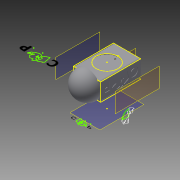
# Autodesk Inventor part: Pieza2
Saved by Autodesk Inventor 2013 (Build 170138000, 138)
## iProperties
Created: 2014-07-03
Part Number: Pieza2
Material: Genérico
Document SubType Name: Chapa
Designer: Administrador
Density: 1 g/cm^3
Sheet Metal Rule: Por defecto_mm
Author: Administrador
Autodesk Inventor part; units mm, degrees
ref_plane "YZ Plane" through (0, 0, 0) normal (1, 0, 0) x (0, 1, 0)
ref_plane "XZ Plane" through (0, 0, 0) normal (0, 1, 0) x (-1, 0, 0)
ref_plane "XY Plane" through (0, 0, 0) normal (0, 0, 1) x (1, 0, 0)
sketch "Boceto1" plane through (0, 0, 0) normal (0, 0, 1) x (1, 0, 0)
  line L0 (-17, 25) -> (17, 25)
  line L1 (17, 25) -> (17, -25)
  line L2 (17, -25) -> (-17, -25)
  line L3 (-17, -25) -> (-17, 25)
  line L4 (17, 25) -> (-17, -25) construction
  line L5 (-17, 25) -> (17, -25) construction
  point P0 (0, 0)
  point P1 (0, 0)
  dimension "d0" = 34
  dimension "d1" = 50
  constraints: 12 end point, 2 midpoint, 2 parallel, 1 coincident, 1 horizontal, 1 perpendicular
  measures "d0" distance of L1.end L2.end
  measures "d1" distance of L0.end L1.end
extrude "Extrusión1" add sketch "Boceto1" along normal mid plane 22
sketch "Boceto2" plane through (-17, -25, 11) normal (0, -1, 0) x (1, 0, 0)
  line L0 (34, 0) -> (34, -22) projected
  line L1 (0, 0) -> (34, 0) projected
  line L2 (0, 0) -> (0, -22) projected
  line L3 (34, -22) -> (0, -22) projected
  line L4 (32, 0) -> (0, -22) construction
  line L5 (0, 0) -> (32, -22) construction
  point P0 (17, -11)
  constraints: 4 end point
ref_plane "Plano de trabajo1" through (1, -25, 11) normal (1, 0, 0) x (0, 0, -1)
sketch "Boceto4" plane through (1, -25, 11) normal (1, 0, 0) x (0, 0, -1)
  arc A0 (62.0687, 50.9812) -> (70.5687, 42.4812) centre (70.5687, 50.9812) ccw
  arc A1 (63.0687, 50.9812) -> (70.5687, 43.4812) centre (70.5687, 50.9812) ccw
  line L0 (70.5687, 50.9812) -> (62.0687, 50.9812)
  line L1 (70.5687, 50.9812) -> (70.5687, 42.4812)
  point P0 (11, 25)
  dimension "d19" = 17
  dimension "d20" = 15
  constraints: 4 end point, 4 point on circle, 2 centre point, 2 point on line
  measures "d19" diameter of A0
  measures "d20" diameter of A1
ref_plane "Plano de trabajo2" through (0, -25, 11) normal (1, 0, 0) x (0, 0, -1)
sketch "Boceto5" plane through (0, -25, 11) normal (1, 0, 0) x (0, 0, -1)
  arc A0 (11, -16.622) -> (28, 0.378) centre (11, 0.378) ccw
  arc A1 (11, -14.622) -> (26, 0.378) centre (11, 0.378) ccw
  line L0 (11, 0.378) -> (11, -19.6766)
  line L1 (11, 0.378) -> (38.473, 0.378)
  point P0 (11, 25)
  dimension "d25" = 34
  dimension "d26" = 30
  constraints: 4 end point, 4 point on circle, 4 point on line, 2 centre point
  measures "d25" diameter of A0
  measures "d26" diameter of A1
revolve "Revolución2" add sketch "Boceto5" angle 360 about axis through (0, -24.622, 0) along (0, -1, 0) contours L0 A1 L1 A0
shell "Vaciado1" thickness 2 removed faces 1 at (5.6667, 25, 3.6667)
sketch "Boceto6" plane through (0, 0, -11) normal (0, 0, -1) x (-1, 0, 0)
  arc A0 (-0.9993, 13.463) -> (0.9993, 13.463) centre (0, 0) ccw
  arc A1 (0.9993, 13.463) -> (-0.9993, 13.463) centre (0, 13.4998) ccw
  dimension "d29" = 27
  dimension "d34" = 2
  constraints: 4 point on circle, 2 centre point
  measures "d29" diameter of A0
  measures "d34" diameter of A1
extrude "Extrusión2" cut sketch "Boceto6" against normal blind 1
sketch "Boceto7" plane through (0, 0, 11) normal (0, 0, 1) x (1, 0, 0)
  arc A0 (-0.9993, 13.463) -> (0.9993, 13.463) centre (0, 0) ccw projected
  arc A1 (0.9993, 13.463) -> (-0.9993, 13.463) centre (0, 13.4998) ccw projected
extrude "Extrusión3" cut sketch "Boceto7" against normal blind 1
hole "Hole2" at (0.5516, 9.7228, -10) direction (0, 0, 1) diameter 2 end through all
sketch "Boceto8" plane through (0, 0, -11) normal (0, 0, -1) x (-1, 0, 0)
  arc A0 (-0.9993, 13.463) -> (0.9993, 13.463) centre (0, 0) ccw projected
  arc A1 (0.9993, 13.463) -> (-0.9993, 13.463) centre (0, 13.4998) ccw projected
  arc A2 (-12.9615, -24.622) -> (-12.956, -25) centre (0, -24.622) ccw projected
  line L0 (-12.9615, -24.622) -> (-10.198, -24.622) projected
  arc A3 (-10.198, -24.622) -> (-10.191, -25) centre (0, -24.622) ccw projected
  line L1 (-10.191, -25) -> (10.191, -25) projected
  arc A4 (10.191, -25) -> (10.198, -24.622) centre (0, -24.622) ccw projected
  line L2 (10.198, -24.622) -> (12.9615, -24.622) projected
  arc A5 (12.956, -25) -> (12.9615, -24.622) centre (0, -24.622) ccw projected
  line L3 (12.956, -25) -> (17, -25) projected
  line L4 (17, -25) -> (17, 25) projected
  line L5 (17, 25) -> (-17, 25) projected
  line L6 (-17, 25) -> (-17, -25) projected
  line L7 (-17, -25) -> (-12.956, -25) projected
sketch "Boceto9" plane through (-15, -23, -9) normal (0, 1, 0) x (1, 0, 0)
  arc A0 (27.9615, 2) -> (2.0385, 2) centre (15, -9) ccw projected
  arc A1 (2.0385, -20) -> (27.9615, -20) centre (15, -9) ccw projected
  circle A2 centre (15, -9) radius 4.05
  point P0 (15, -9)
  dimension "d57" = 8.1
  constraints: 1 centre point
  measures "d57" diameter of A2
extrude "Extrusión4" cut sketch "Boceto9" against normal blind 1
ref_plane "Plano de trabajo3" through (-36.25, -25, 11) normal (-1, 0, 0) x (0, 0, 1)
sketch "Boceto10" plane through (-36.25, -25, 11) normal (-1, 0, 0) x (0, 0, 1)
  line L0 (-17.7826, 33.8086) -> (-14.5363, 27.7029)
  line L1 (-13.9978, 26.6902) -> (-13.9974, 26.6894)
  line L2 (-12.2413, 28.1075) -> (-14.5363, 27.7029)
  line L3 (-11.5169, 27.1267) -> (-14.0003, 26.6889)
  ellipse E0 centre (-9.6601, 27.8136) end of major axis (-7.0347, 26.2904) minor radius 1.6776 (-8.1725, 28.825) -> (-12.2413, 28.1075) ccw
  ellipse E1 centre (-10.8449, 20.7604) end of major axis (-14.0003, 26.6889) minor radius 3.4629 (-13.9978, 26.6902) -> (-7.6919, 14.8305) ccw
  line L4 (-5.4899, 29.298) -> (-8.1725, 28.825)
  line L5 (-4.9509, 28.2844) -> (-7.2786, 27.874)
  line L6 (-4.9509, 28.2844) -> (-3.2498, 25.0851)
  line L7 (-17.7826, 33.8086) -> (-8.7364, 35.4037)
  line L8 (-8.7364, 35.4037) -> (-5.4899, 29.298)
  line L9 (-7.3044, 36.4363) -> (-7.3044, 32.7107) construction
  line L10 (-17.7826, 33.8086) -> (-17.7826, 24.6228) construction
  line L11 (-17.7826, 33.8086) -> (-17.7826, 13.3894) construction
  ellipse E2 centre (-9.6601, 27.8136) end of major axis (-7.0347, 26.2904) minor radius 1.6776 (-11.5169, 27.1267) -> (-7.2786, 27.874) ccw
  ellipse E3 centre (-9.6601, 24.5302) end of major axis (-6.0844, 19.1017) minor radius 3.6119 (-10.4961, 20.1047) -> (-5.6523, 24.6615) ccw
  ellipse E4 centre (-9.0943, 17.4675) end of major axis (-10.4964, 20.1046) minor radius 1.3012 (-10.4961, 20.1047) -> (-7.6919, 14.8305) ccw
  line L12 (-10.4964, 20.1046) -> (-7.6922, 14.8304) construction
  line L13 (-3.2498, 25.0851) -> (-5.6523, 24.6615)
  line L14 (-7.6615, 46.9866) -> (-7.6615, 19.6947) construction
  line L15 (-7.6615, 19.6947) -> (-18.0504, 19.6947) construction
  line L16 (-18.0504, 19.6947) -> (-18.0504, 46.9866) construction
  line L17 (-18.0504, 46.9866) -> (-7.6615, 46.9866) construction
  line L18 (-7.8627, 12.5769) -> (-7.8627, 3.5412) construction
  line L19 (-7.8627, 3.5412) -> (-17.8627, 3.5412) construction
  line L20 (-17.8627, 3.5412) -> (-17.8627, 12.5769) construction
  line L21 (-17.8627, 12.5769) -> (-7.8627, 12.5769) construction
  spline S0 degree 2 poles (-18.0504, 41.6381) (-18.0504, 43.891) (-15.3276, 46.5328) (-12.864, 46.5328) knots 0 0 0 1 2 2 2
  spline S1 degree 2 poles (-12.864, 46.5328) (-10.4897, 46.5328) (-7.6615, 43.8828) (-7.6615, 41.63) knots 0 0 0 1 2 2 2
  spline S2 degree 2 poles (-7.6615, 41.63) (-7.6615, 41.0384) (-7.7992, 40.0822) (-7.9127, 39.6446) knots 0 0 0 1 2 2 2
  spline S3 degree 2 poles (-7.9127, 39.6446) (-8.018, 39.3042) (-8.3665, 38.502) (-8.4961, 38.2508) knots 0 0 0 1 2 2 2
  line L22 (-8.4961, 38.2508) -> (-10.8786, 38.2508)
  line L23 (-10.8786, 38.2508) -> (-10.8786, 38.502)
  spline S4 degree 2 poles (-10.8786, 38.502) (-10.7166, 38.6884) (-10.2627, 39.2394) (-10.0521, 39.5879) knots 0 0 0 1 2 2 2
  spline S5 degree 2 poles (-10.0521, 39.5879) (-9.8333, 39.9363) (-9.5334, 40.771) (-9.5334, 41.2329) knots 0 0 0 1 2 2 2
  spline S6 degree 2 poles (-9.5334, 41.2329) (-9.5334, 41.7759) (-9.8738, 42.6754) (-10.3033, 43.0887) knots 0 0 0 1 2 2 2
  spline S7 degree 2 poles (-10.3033, 43.0887) (-10.6841, 43.4615) (-11.9888, 43.9396) (-12.8721, 43.9396) knots 0 0 0 1 2 2 2
  spline S8 degree 2 poles (-12.8721, 43.9396) (-13.8041, 43.9396) (-15.0764, 43.4452) (-15.4653, 43.0401) knots 0 0 0 1 2 2 2
  spline S9 degree 2 poles (-15.4653, 43.0401) (-15.8462, 42.6511) (-16.1785, 41.6948) (-16.1785, 41.2167) knots 0 0 0 1 2 2 2
  spline S10 degree 2 poles (-16.1785, 41.2167) (-16.1785, 40.7224) (-15.8462, 39.8229) (-15.6436, 39.5149) knots 0 0 0 1 2 2 2
  spline S11 degree 2 poles (-15.6436, 39.5149) (-15.441, 39.1746) (-15.0115, 38.664) (-14.8414, 38.4777) knots 0 0 0 1 2 2 2
  line L24 (-14.8414, 38.4777) -> (-14.8414, 38.2508)
  line L25 (-14.8414, 38.2508) -> (-17.1914, 38.2508)
  spline S12 degree 2 poles (-17.1914, 38.2508) (-17.3211, 38.5263) (-17.6452, 39.2475) (-17.7587, 39.6365) knots 0 0 0 1 2 2 2
  spline S13 degree 2 poles (-17.7587, 39.6365) (-17.9046, 40.1065) (-18.0504, 40.925) (-18.0504, 41.6381) knots 0 0 0 1 2 2 2
  spline S14 degree 2 poles (-11.015, 3.8492) (-11.7119, 3.8492) (-12.9761, 4.2949) (-13.3975, 4.7082) knots 0 0 0 1 2 2 2
  spline S15 degree 2 poles (-13.3975, 4.7082) (-13.6649, 4.9594) (-14.1025, 5.5753) (-14.2565, 5.9399) knots 0 0 0 1 2 2 2
  spline S16 degree 2 poles (-14.2565, 5.9399) (-14.4105, 6.3127) (-14.5888, 7.1798) (-14.5888, 7.7147) knots 0 0 0 1 2 2 2
  line L26 (-14.5888, 7.7147) -> (-14.5888, 9.0275)
  line L27 (-14.5888, 9.0275) -> (-17.8627, 9.0275)
  line L28 (-17.8627, 9.0275) -> (-17.8627, 11.5396)
  line L29 (-17.8627, 11.5396) -> (-7.8627, 11.5396)
  line L30 (-7.8627, 11.5396) -> (-7.8627, 7.6579)
  spline S17 degree 2 poles (-7.8627, 7.6579) (-7.8627, 6.7989) (-8.1787, 5.5429) (-8.5191, 5.0323) knots 0 0 0 1 2 2 2
  spline S18 degree 2 poles (-8.5191, 5.0323) (-8.9, 4.4651) (-10.1479, 3.8492) (-11.015, 3.8492) knots 0 0 0 1 2 2 2
  spline S19 degree 2 poles (-11.0799, 6.4262) (-10.6504, 6.4262) (-10.0426, 6.8313) (-9.9291, 7.1069) knots 0 0 0 1 2 2 2
  spline S20 degree 2 poles (-9.9291, 7.1069) (-9.7752, 7.4634) (-9.7265, 8.1117) (-9.7265, 8.6709) knots 0 0 0 1 2 2 2
  line L31 (-9.7265, 8.6709) -> (-9.7265, 9.0275)
  line L32 (-9.7265, 9.0275) -> (-12.7249, 9.0275)
  line L33 (-12.7249, 9.0275) -> (-12.7249, 8.8492)
  spline S21 degree 2 poles (-12.7249, 8.8492) (-12.7249, 8.5007) (-12.7087, 7.8686) (-12.6682, 7.6336) knots 0 0 0 1 2 2 2
  spline S22 degree 2 poles (-12.6682, 7.6336) (-12.6358, 7.431) (-12.4413, 6.9853) (-12.3197, 6.8638) knots 0 0 0 1 2 2 2
  spline S23 degree 2 poles (-12.3197, 6.8638) (-12.0766, 6.6044) (-11.5337, 6.4262) (-11.0799, 6.4262) knots 0 0 0 1 2 2 2
  point P0 (-11, 25)
  dimension "d63" = 100
  constraints: 28 end point, 2 point on line, 1 equal length, 26 other
  measures "d63" angle of L10 L7
emboss "Repujado2" sketch "Boceto10" operation cut depth 0.5 direction (1, 0, 0)
ref_plane "Plano de trabajo4" through (37.75, -25, 11) normal (1, 0, 0) x (0, 0, -1)
sketch "Boceto11" plane through (37.75, -25, 11) normal (1, 0, 0) x (0, 0, -1)
  line L0 (17.9928, 28.2607) -> (15.6652, 27.8504)
  line L1 (17.4539, 29.2744) -> (14.7713, 28.8014)
  line L2 (14.2074, 35.3801) -> (17.4539, 29.2744)
  ellipse E0 centre (13.2836, 27.79) end of major axis (15.909, 26.2668) minor radius 1.6776 (11.4269, 27.1031) -> (15.6652, 27.8504) ccw
  ellipse E1 centre (13.2836, 27.79) end of major axis (15.909, 26.2668) minor radius 1.6776 (14.7713, 28.8014) -> (10.7025, 28.0839) ccw
  line L3 (15.6393, 36.4127) -> (15.6393, 32.6871) construction
  line L4 (11.4269, 27.1031) -> (8.9435, 26.6653)
  line L5 (10.7025, 28.0839) -> (8.4075, 27.6792)
  line L6 (5.1612, 33.785) -> (8.4075, 27.6792)
  line L7 (5.1612, 33.785) -> (14.2074, 35.3801)
  line L8 (15.2823, 19.6711) -> (4.8933, 19.6711) construction
  line L9 (4.8933, 46.9629) -> (15.2823, 46.9629) construction
  line L10 (15.2823, 46.9629) -> (15.2823, 19.6711) construction
  line L11 (4.8933, 19.6711) -> (4.8933, 46.9629) construction
  line L12 (8.9459, 26.6666) -> (8.9464, 26.6658)
  line L13 (17.9928, 28.2607) -> (19.6939, 25.0615)
  line L14 (19.6939, 25.0615) -> (17.2915, 24.6379)
  ellipse E2 centre (13.2836, 24.5066) end of major axis (16.8594, 19.0781) minor radius 3.6119 (12.4477, 20.0811) -> (17.2915, 24.6379) ccw
  line L15 (12.4474, 20.0809) -> (15.2516, 14.8068) construction
  ellipse E3 centre (13.8495, 17.4439) end of major axis (12.4474, 20.0809) minor radius 1.3012 (12.4477, 20.0811) -> (15.2518, 14.8069) ccw
  ellipse E4 centre (12.0989, 20.7367) end of major axis (8.9435, 26.6653) minor radius 3.4628 (8.9459, 26.6666) -> (15.2518, 14.8069) ccw
  line L16 (5.0811, 12.5533) -> (15.0811, 12.5533) construction
  line L17 (15.0811, 12.5533) -> (15.0811, 3.5176) construction
  line L18 (15.0811, 3.5176) -> (5.0811, 3.5176) construction
  line L19 (5.0811, 3.5176) -> (5.0811, 12.5533) construction
  spline S0 degree 2 poles (4.8933, 41.6145) (4.8933, 43.8673) (7.6162, 46.5091) (10.0797, 46.5091) knots 0 0 0 1 2 2 2
  spline S1 degree 2 poles (10.0797, 46.5091) (12.4541, 46.5091) (15.2823, 43.8592) (15.2823, 41.6064) knots 0 0 0 1 2 2 2
  spline S2 degree 2 poles (15.2823, 41.6064) (15.2823, 41.0148) (15.1446, 40.0586) (15.0311, 39.621) knots 0 0 0 1 2 2 2
  spline S3 degree 2 poles (15.0311, 39.621) (14.9258, 39.2806) (14.5773, 38.4783) (14.4476, 38.2271) knots 0 0 0 1 2 2 2
  line L20 (14.4476, 38.2271) -> (12.0651, 38.2271)
  line L21 (12.0651, 38.2271) -> (12.0651, 38.4783)
  spline S4 degree 2 poles (12.0651, 38.4783) (12.2272, 38.6647) (12.681, 39.2158) (12.8917, 39.5642) knots 0 0 0 1 2 2 2
  spline S5 degree 2 poles (12.8917, 39.5642) (13.1105, 39.9127) (13.4104, 40.7474) (13.4104, 41.2093) knots 0 0 0 1 2 2 2
  spline S6 degree 2 poles (13.4104, 41.2093) (13.4104, 41.7522) (13.07, 42.6518) (12.6405, 43.0651) knots 0 0 0 1 2 2 2
  spline S7 degree 2 poles (12.6405, 43.0651) (12.2596, 43.4378) (10.9549, 43.9159) (10.0716, 43.9159) knots 0 0 0 1 2 2 2
  spline S8 degree 2 poles (10.0716, 43.9159) (9.1397, 43.9159) (7.8674, 43.4216) (7.4784, 43.0164) knots 0 0 0 1 2 2 2
  spline S9 degree 2 poles (7.4784, 43.0164) (7.0976, 42.6275) (6.7653, 41.6712) (6.7653, 41.1931) knots 0 0 0 1 2 2 2
  spline S10 degree 2 poles (6.7653, 41.1931) (6.7653, 40.6988) (7.0976, 39.7993) (7.3001, 39.4913) knots 0 0 0 1 2 2 2
  spline S11 degree 2 poles (7.3001, 39.4913) (7.5027, 39.151) (7.9322, 38.6404) (8.1024, 38.454) knots 0 0 0 1 2 2 2
  line L22 (8.1024, 38.454) -> (8.1024, 38.2271)
  line L23 (8.1024, 38.2271) -> (5.7523, 38.2271)
  spline S12 degree 2 poles (5.7523, 38.2271) (5.6227, 38.5027) (5.2985, 39.2239) (5.1851, 39.6129) knots 0 0 0 1 2 2 2
  spline S13 degree 2 poles (5.1851, 39.6129) (5.0392, 40.0829) (4.8933, 40.9014) (4.8933, 41.6145) knots 0 0 0 1 2 2 2
  spline S14 degree 2 poles (11.9287, 3.8255) (11.2318, 3.8255) (9.9676, 4.2713) (9.5462, 4.6845) knots 0 0 0 1 2 2 2
  spline S15 degree 2 poles (9.5462, 4.6845) (9.2788, 4.9358) (8.8412, 5.5516) (8.6872, 5.9163) knots 0 0 0 1 2 2 2
  spline S16 degree 2 poles (8.6872, 5.9163) (8.5333, 6.2891) (8.355, 7.1562) (8.355, 7.691) knots 0 0 0 1 2 2 2
  line L24 (8.355, 7.691) -> (8.355, 9.0038)
  line L25 (8.355, 9.0038) -> (5.0811, 9.0038)
  line L26 (5.0811, 9.0038) -> (5.0811, 11.516)
  line L27 (5.0811, 11.516) -> (15.0811, 11.516)
  line L28 (15.0811, 11.516) -> (15.0811, 7.6343)
  spline S17 degree 2 poles (15.0811, 7.6343) (15.0811, 6.7753) (14.765, 5.5192) (14.4247, 5.0087) knots 0 0 0 1 2 2 2
  spline S18 degree 2 poles (14.4247, 5.0087) (14.0438, 4.4414) (12.7958, 3.8255) (11.9287, 3.8255) knots 0 0 0 1 2 2 2
  spline S19 degree 2 poles (11.8639, 6.4025) (12.2934, 6.4025) (12.9012, 6.8077) (13.0146, 7.0832) knots 0 0 0 1 2 2 2
  spline S20 degree 2 poles (13.0146, 7.0832) (13.1686, 7.4398) (13.2172, 8.0881) (13.2172, 8.6473) knots 0 0 0 1 2 2 2
  line L29 (13.2172, 8.6473) -> (13.2172, 9.0038)
  line L30 (13.2172, 9.0038) -> (10.2189, 9.0038)
  line L31 (10.2189, 9.0038) -> (10.2189, 8.8255)
  spline S21 degree 2 poles (10.2189, 8.8255) (10.2189, 8.4771) (10.2351, 7.845) (10.2756, 7.61) knots 0 0 0 1 2 2 2
  spline S22 degree 2 poles (10.2756, 7.61) (10.308, 7.4074) (10.5025, 6.9617) (10.624, 6.8401) knots 0 0 0 1 2 2 2
  spline S23 degree 2 poles (10.624, 6.8401) (10.8671, 6.5808) (11.4101, 6.4025) (11.8639, 6.4025) knots 0 0 0 1 2 2 2
  point P0 (11, 25)
  point P1 (11.9438, 24.9764)
  point P2 (5.1612, 24.5992)
  point P3 (5.1612, 13.3657)
  constraints: 24 end point, 2 point on line, 26 other
emboss "Repujado3" sketch "Boceto11" operation cut depth 0.5 direction (-1, 0, 0)
sketch "Boceto12" plane through (0, 0, 11) normal (0, 0, 1) x (1, 0, 0)
  arc A0 (0.9993, 13.463) -> (-0.9993, 13.463) centre (0, 13.4998) ccw projected
  arc A1 (-0.9993, 13.463) -> (0.9993, 13.463) centre (0, 0) ccw projected
  arc A2 (12.956, -25) -> (12.9615, -24.622) centre (0, -24.622) ccw projected
  line L0 (12.956, -25) -> (17, -25) projected
  line L1 (17, -25) -> (17, 25) projected
  line L2 (17, 25) -> (-17, 25) projected
  line L3 (-17, 25) -> (-17, -25) projected
  line L4 (-17, -25) -> (-12.956, -25) projected
  arc A3 (-12.9615, -24.622) -> (-12.956, -25) centre (0, -24.622) ccw projected
  line L5 (-12.9615, -24.622) -> (-10.198, -24.622) projected
  arc A4 (-10.198, -24.622) -> (-10.191, -25) centre (0, -24.622) ccw projected
  line L6 (-10.191, -25) -> (10.191, -25) projected
  arc A5 (10.191, -25) -> (10.198, -24.622) centre (0, -24.622) ccw projected
  line L7 (10.198, -24.622) -> (12.9615, -24.622) projected
  ellipse E0 centre (-46.8772, -38.1339) end of major axis (-48.4004, -40.7593) minor radius 1.6776 (-47.564, -36.2772) -> (-46.8168, -40.5154) ccw
  ellipse E1 centre (-50.1606, -38.1339) end of major axis (-55.589, -41.7097) minor radius 3.6119 (-54.5861, -37.2979) -> (-50.0293, -42.1417) ccw
  ellipse E2 centre (-46.8772, -38.1339) end of major axis (-48.4004, -40.7593) minor radius 1.6776 (-45.8658, -39.6215) -> (-46.5832, -35.5528) ccw
  line L8 (-48.0006, -33.7962) -> (-48.0014, -33.7966)
  line L9 (-47.564, -36.2772) -> (-48.0019, -33.7938)
  ellipse E3 centre (-53.9304, -36.9491) end of major axis (-48.0019, -33.7938) minor radius 3.4628 (-48.0006, -33.7962) -> (-59.8602, -40.1021) ccw
  line L10 (-54.5862, -37.2977) -> (-59.8604, -40.1019) construction
  ellipse E4 centre (-57.2233, -38.6998) end of major axis (-54.5862, -37.2977) minor radius 1.3012 (-54.5861, -37.2979) -> (-59.8602, -40.1021) ccw
  line L11 (-49.6057, -44.5442) -> (-50.0293, -42.1417)
  line L12 (-46.4064, -42.8431) -> (-46.8168, -40.5154)
  line L13 (-45.3928, -42.3041) -> (-45.8658, -39.6215)
  line L14 (-46.4064, -42.8431) -> (-49.6057, -44.5442)
  line L15 (-62.1139, -29.9314) -> (-62.1139, -39.9314) construction
  line L16 (-62.1139, -39.9314) -> (-71.1496, -39.9314) construction
  line L17 (-71.1496, -39.9314) -> (-71.1496, -29.9314) construction
  line L18 (-71.1496, -29.9314) -> (-62.1139, -29.9314) construction
  line L19 (-39.2871, -39.0577) -> (-45.3928, -42.3041)
  line L20 (-38.2545, -40.4896) -> (-41.9801, -40.4896) construction
  line L21 (-54.9961, -40.1326) -> (-54.9961, -29.7436) construction
  line L22 (-27.7042, -40.1326) -> (-54.9961, -40.1326) construction
  line L23 (-46.5832, -35.5528) -> (-46.9879, -33.2578)
  line L24 (-40.8822, -30.0114) -> (-39.2871, -39.0577)
  line L25 (-40.8822, -30.0114) -> (-46.9879, -33.2578)
  line L26 (-27.7042, -29.7436) -> (-27.7042, -40.1326) construction
  line L27 (-54.9961, -29.7436) -> (-27.7042, -29.7436) construction
  point P0 (-49.6672, -35.8503)
  point P1 (-49.6908, -36.794)
  point P2 (-50.0679, -30.0114)
  point P3 (-61.3014, -30.0114)
  constraints: 24 end point, 2 point on line, 26 other
ref_plane "Plano de trabajo5" through (0, 0, -39) normal (0, 0, -1) x (-1, 0, 0)
sketch "Boceto13" plane through (0, 0, -39) normal (0, 0, -1) x (-1, 0, 0)
  line L0 (13.1941, -26.6662) -> (13.1941, -32.7957) construction
  line L1 (13.1941, -32.7957) -> (-2.9082, -32.7957) construction
  line L2 (-2.9082, -32.7957) -> (-2.9082, -26.6662) construction
  line L3 (-2.9082, -26.6662) -> (13.1941, -26.6662) construction
  line L4 (5.4191, -26.8243) -> (1.8167, -28.7396)
  line L5 (6.3602, -32.1615) -> (2.7578, -34.077)
  line L6 (6.9694, -33.0064) -> (4.7713, -33.0064) construction
  line L7 (5.4191, -26.8243) -> (6.3602, -32.1615)
  line L8 (-7.1077, -26.777) -> (-7.1077, -32.677) construction
  line L9 (-7.1077, -32.677) -> (-12.4387, -32.677) construction
  line L10 (-12.4387, -32.677) -> (-12.4387, -26.777) construction
  line L11 (-12.4387, -26.777) -> (-7.1077, -26.777) construction
  line L12 (1.2192, -29.0573) -> (1.2187, -29.0575)
  ellipse E0 centre (-2.2794, -30.9175) end of major axis (1.2184, -29.0558) minor radius 2.0431 (1.2192, -29.0573) -> (-5.778, -32.7777) ccw
  line L13 (-2.6663, -31.1231) -> (-5.7781, -32.7776) construction
  ellipse E1 centre (-4.2222, -31.9504) end of major axis (-2.6663, -31.1231) minor radius 0.7677 (-2.6662, -31.1233) -> (-5.778, -32.7777) ccw
  line L14 (2.0554, -30.0936) -> (1.8167, -28.7396)
  line L15 (2.7578, -34.077) -> (2.4787, -32.4942)
  line L16 (1.4768, -30.521) -> (1.2184, -29.0558)
  line L17 (2.1598, -34.3949) -> (1.9176, -33.0216)
  ellipse E2 centre (1.882, -31.6165) end of major axis (0.9833, -33.1655) minor radius 0.9898 (1.4768, -30.521) -> (1.9176, -33.0216) ccw
  line L18 (2.1598, -34.3949) -> (0.2722, -35.3986)
  line L19 (0.2722, -35.3986) -> (0.0223, -33.9811)
  ellipse E3 centre (-0.0552, -31.6165) end of major axis (-3.258, -33.7262) minor radius 2.131 (-2.6662, -31.1233) -> (0.0223, -33.9811) ccw
  ellipse E4 centre (1.882, -31.6165) end of major axis (0.9833, -33.1655) minor radius 0.9898 (2.4787, -32.4942) -> (2.0554, -30.0936) ccw
  point P0 (0, 0)
  point P1 (0.2359, -30.2692)
  point P2 (0.222, -30.826)
  point P3 (-0.0006, -26.8243)
  point P4 (-6.6283, -26.8243)
  constraints: 24 end point, 2 point on line, 26 other
fillet "Empalme3" radius 2 4 edges at (17, 0, -11) (17, 0, 11) (-17, 0, 11) (-17, 0, -11)
sketch "Boceto14" plane through (0, 0, -11) normal (0, 0, -1) x (-1, 0, 0)
  line L0 (12.7692, 17.6804) -> (-28.7739, 17.6804) construction
  line L1 (-28.7739, 17.6804) -> (-28.7739, 23.8649) construction
  line L2 (-28.7739, 23.8649) -> (12.7692, 23.8649) construction
  line L3 (12.7692, 23.8649) -> (12.7692, 17.6804) construction
  constraints: 2 other
feature "Repujado7" [suppressed]
equation "\"Radiodetransición\" = Radio_pliegue"
equation "\"Radio_pliegue\" = Grosor"
equation "\"Anchura_desahogo_plegado\" = Grosor"
equation "\"Profundidad_desahogo_plegado\" = 0.5 * Grosor"
equation "\"Tamaño_destalonado\" = 4 * Grosor"
equation "\"Remanente_mínimo\" = 2 * Grosor"
equation "\"Tamaño_de_radio_de_Jacobi\" = Radio_pliegue"
equation "\"TamañoSeparación\" = Grosor"
equation "\"Grosor\" = 0.5"
